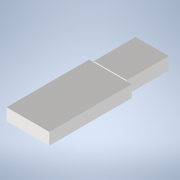
# Autodesk Inventor part: TTLUSB
Saved by Autodesk Inventor 2022 (Build 260153000, 153)
## iProperties
Created: 2021-11-04
Part Number: TTLUSB
Material: Generisch
Document SubType Name: Modeling
Designer: lukas
Density: 1 g/cm^3
Appearance: Vorgabe
Author: lukas
Autodesk Inventor part; units mm, degrees
ref_plane "YZ Plane" through (0, 0, 0) normal (1, 0, 0) x (0, 1, 0)
ref_plane "XZ Plane" through (0, 0, 0) normal (0, 1, 0) x (-1, 0, 0)
ref_plane "XY Plane" through (0, 0, 0) normal (0, 0, 1) x (1, 0, 0)
sketch "Skizze1" plane through (0, 0, 0) normal (0, 1, 0) x (-1, 0, 0)
  line L0 (0, 0) -> (-15.5, 0)
  line L1 (-15.5, 0) -> (-15.5, -30)
  line L2 (-15.5, -30) -> (0, -30)
  line L3 (0, -30) -> (0, 0)
  dimension "d0" = 15.5
  dimension "d1" = 30
  constraints: 8 end point, 2 parallel, 1 horizontal, 1 perpendicular
  measures "d0" distance of L2.end L1.end
  measures "d1" distance of L1.end L0.end
extrude "Extrusion1" add sketch "Skizze1" along normal blind 4.4
sketch "Skizze2" plane through (15.5, 0, -30) normal (0, 0, -1) x (-1, 0, 0)
  line L0 (1.75, 4.8) -> (13.75, 4.8)
  line L1 (13.75, 4.8) -> (13.75, 0.2)
  line L2 (13.75, 0.2) -> (1.75, 0.2)
  line L3 (1.75, 0.2) -> (1.75, 4.8)
  line L4 (0, 0) -> (15.5, 0) projected
  line L5 (15.5, 0) -> (15.5, 4.4) projected
  line L6 (0, 4.4) -> (15.5, 4.4) projected
  line L7 (0, 0) -> (0, 4.4) projected
  point P0 (7.75, 0.2)
  point P1 (7.75, 0)
  dimension "d4" = 12
  dimension "d5" = 4.6
  dimension "d6" = 0.2
  constraints: 8 end point, 2 midpoint, 2 parallel, 1 horizontal, 1 perpendicular, 1 vertical alignment
  measures "d4" distance of L1.end L2.end
  measures "d5" distance of L0.end L1.end
  measures "d6" distance between parallel lines of L4 L2
extrude "Extrusion2" add sketch "Skizze2" along normal blind 15.2 contours L0 L1 L6 L3 | L6 L1 L2 L3
